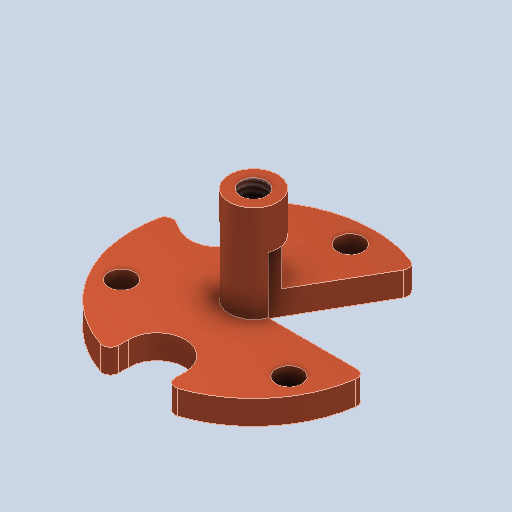
# Autodesk Inventor part: FrameSupport-Flange-Slit
Saved by Autodesk Inventor 2026 (Build 300175050, 175E)
## iProperties
Created: 2023-08-18
Part Number: FrameSupport-Flange-Slit
Material: Copper
Document SubType Name: Modeling
Designer: schanen
Density: 8.94 g/cm^3
Appearance: Copper - Satin
Author: schanen
Autodesk Inventor part; units mm, degrees
ref_plane "YZ Plane" through (0, 0, 0) normal (1, 0, 0) x (0, 1, 0)
ref_plane "XZ Plane" through (0, 0, 0) normal (0, 1, 0) x (-1, 0, 0)
ref_plane "XY Plane" through (0, 0, 0) normal (0, 0, 1) x (1, 0, 0)
sketch "Sketch1" plane through (0, 0, 0) normal (0, 1, 0) x (-1, 0, 0)
  circle A0 centre (0, 0) radius 15
  dimension "d0" = 30
  constraints: 1 centre point, 1 coincident
  measures "d0" diameter of A0
extrude "Extrusion1" add sketch "Sketch1" along normal blind 3
sketch "Sketch2" plane through (0, 3, 0) normal (0, 1, 0) x (1, 0, 0)
  circle A0 centre (0, 0) radius 12 construction
  point P0 (0, 12)
  point P1 (-10.3923, -6)
  point P2 (10.3923, -6)
  dimension "d3" = 24
  dimension "d4" = 120
  constraints: 3 point on circle, 1 centre point, 1 coincident, 1 horizontal alignment, 1 vertical alignment
  measures "d3" diameter of A0
hole "Hole1" at (0, 3, -12) at (-10.3923, 3, 6) at (10.3923, 3, 6) direction (0, -1, 0) diameter 3.2 end through all
sketch "Sketch4" plane through (0, 3, 0) normal (0, 1, 0) x (1, 0, 0)
  circle A0 centre (0, -12) radius 3.5
  circle A1 centre (0, 0) radius 15 projected
  arc A2 (-3.5, -14.586) -> (3.5, -14.586) centre (0, 0) ccw
  line L0 (3.5, -12) -> (3.5, -14.586)
  line L1 (-3.5, -12) -> (-3.5, -14.586)
  dimension "d12" = 7
  dimension "d13" = 12
  constraints: 6 point on circle, 4 end point, 2 centre point, 2 tangent, 2 vertical, 1 coincident, 1 vertical alignment
  measures "d12" diameter of A0
  measures "d13" distance of point (0, 0) A0.centre
extrude "Extrusion2" cut sketch "Sketch4" against normal through all contours A0 A1 | L0 A1 A0 | A0 A1 L1 picked at (0.1406, -12.8318)
pattern_circular "Circular Pattern1" count 3 over 360 about axis through (0, 0, 0) along (0, 1, 0) of "Extrusion2"
sketch "Sketch6" plane through (0, 3, 0) normal (0, 1, 0) x (1, 0, 0)
  circle A0 centre (0, 0) radius 3
  dimension "d24" = 6
  constraints: 1 centre point, 1 coincident
  measures "d24" diameter of A0
extrude "Extrusion4" add sketch "Sketch6" along normal blind 12
sketch "Sketch7" plane through (0, 0, 0) normal (0, -1, 0) x (1, 0, 0)
  line L0 (-1.5, 0) -> (63.9289, 0) construction
  line L1 (0, -1.5) -> (62.4289, -1.5)
  line L2 (62.4289, 1.5) -> (0, 1.5)
  arc A0 (0, 1.5) -> (0, -1.5) centre (0, 0) ccw
  arc A1 (62.4289, -1.5) -> (62.4289, 1.5) centre (62.4289, 0) ccw
  point P0 (31.2144, 0)
  dimension "d27" = 3
  constraints: 8 end point, 6 point on circle, 4 tangent, 2 centre point, 2 point on line, 1 coincident, 1 horizontal, 1 midpoint, 1 parallel
  measures "d27" diameter of A1
extrude "Extrusion5" [suppressed]
sketch "Sketch8" plane through (0, 15, 0) normal (0, 1, 0) x (1, 0, 0)
  point P0 (0, 0)
  point P1 (0, 0)
  constraints: 1 coincident
hole "Hole2" at (0, 15, 0) direction (0, -1, 0) diameter 3.242 end through all thread size "M4x0.7" class "6H" standard "ANSI Metric M Profile"
sketch "Sketch9" plane through (0, 0, 0) normal (0, -1, 0) x (1, 0, 0)
  arc A0 (12.1423, -2.9689) -> (8.6423, -9.0311) centre (10.3923, -6) ccw projected
  line L0 (0, 0) -> (10.3923, -6) construction
  line L1 (0, 0) -> (9.8835, -17.1187) construction
  line L2 (0, 0) -> (17.8778, 0) construction
  line L3 (19.4334, 1) -> (1.2758, 1)
  circle A1 centre (0, 0) radius 1.621 projected
  line L4 (-0.2281, -1.6049) -> (7.499, -14.9886)
  arc A2 (-10.8818, -10.3241) -> (10.8818, -10.3241) centre (0, 0) ccw projected
  arc A3 (14.3818, -4.2619) -> (3.5, 14.586) centre (0, 0) ccw projected
  arc A4 (6.6173, -13.4615) -> (14.9666, 1) centre (0, 0) ccw
  point P0 (10.8818, -10.3241)
  point P1 (14.3818, -4.2619)
  dimension "d37" = 30
  dimension "d38" = 30
  dimension "d39" = 1
  dimension "d40" = 1
  constraints: 10 end point, 6 point on circle, 2 horizontal, 2 parallel, 2 point on line, 1 centre point, 1 coincident
  measures "d37" angle of L2 L0
  measures "d38" angle of L1 L0
  measures "d39" distance between parallel lines of L2 L3
  measures "d40" distance between parallel lines of L4 L1
extrude "Extrusion6" cut sketch "Sketch9" against normal blind 10 contours A3 A4 A2 L4 A1 L3
fillet "Fillet1" radius 1 6 edges at (14.9666, 1.5, 1) (6.6173, 1.5, -13.4615) (-3.5, 1.5, 14.586) (3.5, 1.5, 14.586) (-14.3818, 1.5, -4.2619) (-10.8818, 1.5, -10.3241)
equation "\"d38\" = d37"
equation "\"d40\" = d39"
body "Solid1"
